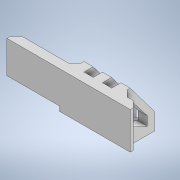
# Autodesk Inventor part: StandBtn
Saved by Autodesk Inventor 2020.1 (Build 241239000, 239)
## iProperties
Created: 2019-09-05
Part Number: StandBtn
Material: Generic
Document SubType Name: Modeling
Designer: matteo.spadetto-1
Density: 1 g/cm^3
Appearance: Default
Author: matteo.spadetto-1
Autodesk Inventor part; units mm, degrees
ref_plane "YZ Plane" through (0, 0, 0) normal (1, 0, 0) x (0, 1, 0)
ref_plane "XZ Plane" through (0, 0, 0) normal (0, 1, 0) x (-1, 0, 0)
ref_plane "XY Plane" through (0, 0, 0) normal (0, 0, 1) x (1, 0, 0)
sketch "Sketch1" plane through (0, 0, 0) normal (0, 0, 1) x (1, 0, 0)
  line L0 (0, 0) -> (5, 0)
  line L1 (5, 0) -> (19, 0)
  line L2 (19, 0) -> (33, 0)
  line L3 (33, 0) -> (28, 0)
  circle A0 centre (5, 0) radius 5
  circle A1 centre (19, 0) radius 5
  circle A2 centre (33, 0) radius 5
  line L4 (0, 0) -> (-1, 0)
  line L5 (38, 0) -> (39, 0)
  line L6 (33, -5) -> (33, -6)
  line L7 (-1, 6) -> (39, 6)
  line L8 (39, 6) -> (39, -6)
  line L9 (39, -6) -> (-1, -6)
  line L10 (-1, -6) -> (-1, 6)
  dimension "d0" = 5
  dimension "d1" = 14
  dimension "d2" = 14
  dimension "d3" = 5
  dimension "d4" = 10
  dimension "d5" = 10
  dimension "d6" = 10
  dimension "d9" = 1
  dimension "d10" = 1
  dimension "d11" = 1
  constraints: 22 end point, 4 horizontal, 3 centre point, 3 coincident, 3 point on line, 2 parallel, 2 point on circle, 1 perpendicular, 1 vertical
  measures "d0" distance of L0.start L0.end
  measures "d1" distance of L0.end L1.end
  measures "d2" distance of L1.end L2.end
  measures "d3" distance of L2.end L3.end
  measures "d4" diameter of A0
  measures "d5" diameter of A1
  measures "d6" diameter of A2
  measures "d9" distance of L0.start L4.end
  measures "d10" distance of L5.start L5.end
  measures "d11" distance of L6.start L6.end
extrude "Extrusion1" add sketch "Sketch1" along normal blind 3
sketch "Sketch2" plane through (-1, 6, 0) normal (0, 1, 0) x (1, 0, 0)
  line L0 (0, -3) -> (40, -3) projected
  line L1 (19, 2) -> (19, 12)
  line L2 (19, 12) -> (34, 12)
  line L3 (34, 12) -> (34, 2)
  line L4 (34, 0) -> (19, 0)
  line L5 (40, 0) -> (36, 0)
  line L6 (36, 0) -> (34, 2)
  line L7 (0, 0) -> (40, 0) projected
  line L8 (17, 0) -> (0, 0)
  line L9 (19, 2) -> (17, 0)
  line L10 (36, 0) -> (17, 0)
  point P0 (1, 0)
  dimension "d16" = 12
  dimension "d17" = 2
  dimension "d19" = 2
  dimension "d20" = 2
  constraints: 18 end point, 5 point on line, 2 collinear, 2 perpendicular, 1 parallel, 1 vertical
  measures "d16" distance of L4.end L1.end
  measures "d17" distance of L5.end point (34, 0)
  measures "d19" distance of L1.start L4.end
  measures "d20" distance of L8.start L4.end
extrude "Extrusion2" add sketch "Sketch2" against normal blind 16
sketch "Sketch3" plane through (-1, 6, 3) normal (0, 1, 0) x (1, 0, 0)
  line L0 (34, 5) -> (34, 15) projected
  line L1 (34, 5) -> (34, -8.5215)
  line L2 (34, -8.5215) -> (31, -8.5215)
  line L3 (31, -8.5215) -> (28, -8.5215)
  line L4 (28, -8.5215) -> (25, -8.5215)
  line L5 (25, -8.5215) -> (22, -8.5215)
  line L6 (22, -8.5215) -> (19, -8.5215)
  line L7 (34, 5) -> (34, 3)
  line L8 (17, 3) -> (36, 3) projected
  line L9 (31, 3) -> (31, 15)
  line L10 (34, 15) -> (19, 15) projected
  line L11 (31, 15) -> (34, 15)
  line L12 (34, 15) -> (34, 5)
  line L13 (34, 3) -> (31, 3)
  line L14 (31, 3) -> (28, 3)
  line L15 (28, 3) -> (28, 15)
  line L16 (28, 15) -> (31, 15)
  line L17 (28, 3) -> (25, 3)
  line L18 (25, 3) -> (25, 15)
  line L19 (25, 15) -> (28, 15)
  line L20 (25, 3) -> (22, 3)
  line L21 (22, 3) -> (22, 15)
  line L22 (22, 15) -> (25, 15)
  line L23 (22, 3) -> (19, 3)
  line L24 (19, 15) -> (19, 5) projected
  line L25 (19, 3) -> (19, 15)
  line L26 (19, 15) -> (22, 15)
  point P0 (1, 3)
  dimension "d27" = 3
  dimension "d28" = 3
  dimension "d29" = 3
  dimension "d30" = 3
  dimension "d31" = 3
  constraints: 46 end point, 14 point on line, 8 perpendicular, 3 collinear, 1 horizontal, 1 parallel, 1 vertical
  measures "d27" distance of L1.end L2.end
  measures "d28" distance of L2.end L3.end
  measures "d29" distance of L3.end L4.end
  measures "d30" distance of L4.end L5.end
  measures "d31" distance of L5.end L6.end
extrude "Extrusion3" cut sketch "Sketch3" against normal blind 15 contours L9 L8 L15 L10 | L18 L8 L21 L10
sketch "Sketch4" plane through (39, -6, 0) normal (1, 0, 0) x (0, 0, -1)
  line L0 (2, 12) -> (2, -4) projected
  line L1 (0, 0) -> (2, -4)
  line L2 (2, -4) -> (2, 0)
  line L3 (0, 0) -> (2, 0)
  line L4 (2, 12) -> (2, 10)
  line L5 (12, -3) -> (2, 10)
  line L6 (2, 0) -> (2, 1.5)
  line L7 (2, 10) -> (2, 1.5)
  line L8 (2, 1.5) -> (12, -3)
  line L9 (2, 12) -> (12, 12) projected
  line L10 (12, 12) -> (12, -4) projected
  line L11 (12, -3) -> (12, -1)
  line L12 (12, -1) -> (12, 0)
  line L13 (12, 0) -> (3, 12)
  line L14 (2, 12) -> (3, 12)
  line L15 (3, 12) -> (12, 12)
  line L16 (12, 12) -> (12, 0)
  line L17 (0, 0) -> (0, -3) projected
  line L18 (0, 0) -> (0, -4) projected
  line L19 (0, 0) -> (0, -4)
  line L20 (2, -4) -> (0, -4) projected
  line L21 (0, -4) -> (2, -4)
  line L22 (8.5385, 1.5) -> (8.5385, -1.4423)
  point P0 (0, 6)
  dimension "d34" = 2
  dimension "d35" = 1.5
  dimension "d37" = 2
  dimension "d38" = 1
  constraints: 34 end point, 9 point on line, 3 collinear, 3 perpendicular, 2 vertical
  measures "d34" distance of L0.start L4.end
  measures "d35" distance of L2.end L6.end
  measures "d37" distance of L11.start L11.end
  measures "d38" distance of L11.end L12.end
extrude "Extrusion5" cut sketch "Sketch4" against normal blind 25 contours L5 L22 L8 L0 | L9 L10 L13 | L20 L18 L17 L1
chamfer "Chamfer1" distance 2 angle 45 1 edges at (-1, 0, 0)
chamfer "Chamfer2" distance 2 angle 45 1 edges at (39, 0, 0)
sketch "Sketch5" plane through (33, 6, -2) normal (1, 0, 0) x (0, 0, -1)
  line L0 (10, -16) -> (0, -16) projected
  line L1 (10, -16) -> (8.9, -16)
  line L2 (8.9, -16) -> (8.9, -9)
  line L3 (8.9, -9) -> (10, -9)
  line L4 (10, -9) -> (10, -16)
  point P0 (-2, -6)
  dimension "d49" = 1.1
  dimension "d50" = 7
  constraints: 8 end point, 2 parallel, 1 horizontal, 1 perpendicular
  measures "d49" distance of L2.end L3.end
  measures "d50" distance of L3.end L0.start
extrude "Extrusion6" cut sketch "Sketch5" against normal blind 15
sketch "Sketch6" plane through (0, 0, 0) normal (0, 0, -1) x (-1, 0, 0)
  line L0 (-1, -6) -> (-16, -6) projected
  line L1 (1, 6) -> (1, -6) projected
  line L2 (-16, -6) -> (1, -6)
  line L3 (1, -6) -> (1, -4.5)
  line L4 (1, -4.5) -> (-16, -4.5)
  line L5 (-16, -4.5) -> (-16, -6)
  point P0 (0, 0)
  dimension "d53" = 1.5
  constraints: 8 end point, 2 parallel, 1 horizontal, 1 perpendicular, 1 point on line
  measures "d53" distance of L3.end L2.end
extrude "Extrusion7" cut sketch "Sketch6" against normal blind 10
equation "\"d20\" = d19"
body "Solid1"
